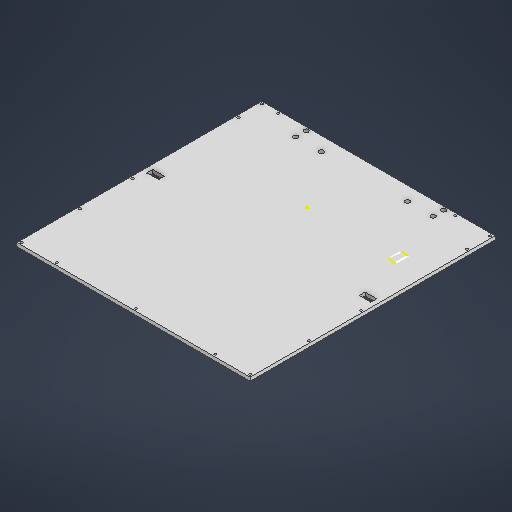
# Autodesk Inventor part: DesignBawahRobot
Saved by Autodesk Inventor 2026.1 (Build 301233020, 233B)
## iProperties
Created: 2025-10-17
Part Number: DesignBawahRobot
Material: Generic
Document SubType Name: Modeling
Designer: FrianVex
Density: 1 g/cm^3
Appearance: Default
Author: FrianVex
Autodesk Inventor part; units mm, degrees
ref_plane "YZ Plane" through (0, 0, 0) normal (1, 0, 0) x (0, 1, 0)
ref_plane "XZ Plane" through (0, 0, 0) normal (0, 1, 0) x (-1, 0, 0)
ref_plane "XY Plane" through (0, 0, 0) normal (0, 0, 1) x (1, 0, 0)
sketch "Sketch1" plane through (0, 0, 0) normal (0, 1, 0) x (-1, 0, 0)
  line L0 (-101.0152, -60.2536) -> (98.9848, -60.2536)
  line L1 (98.9848, -60.2536) -> (98.9848, 149.7464)
  line L2 (98.9848, 149.7464) -> (-101.0152, 149.7464)
  line L3 (-101.0152, 149.7464) -> (-101.0152, -60.2536)
  line L4 (-101.0152, -60.2536) -> (98.9848, 149.7464) construction
  line L5 (98.9848, -60.2536) -> (-101.0152, 149.7464) construction
  line L6 (-65.0152, -60.2536) -> (62.9848, -60.2536)
  line L7 (62.9848, -60.2536) -> (62.9848, -45.2536)
  line L8 (62.9848, -45.2536) -> (-65.0152, -45.2536)
  line L9 (-65.0152, -45.2536) -> (-65.0152, -60.2536)
  line L10 (98.9848, -35.2536) -> (76.9848, -35.2536)
  line L11 (76.9848, -35.2536) -> (76.9848, 34.7464)
  line L12 (76.9848, 34.7464) -> (98.9848, 34.7464)
  line L13 (98.9848, 34.7464) -> (98.9848, -35.2536)
  line L14 (-101.0152, -35.2536) -> (-79.0152, -35.2536)
  line L15 (-79.0152, -35.2536) -> (-79.0152, 34.7464)
  line L16 (-79.0152, 34.7464) -> (-101.0152, 34.7464)
  line L17 (-101.0152, 34.7464) -> (-101.0152, -35.2536)
  line L18 (84.9848, 37.2464) -> (94.9848, 37.2464)
  line L19 (94.9848, 37.2464) -> (94.9848, 42.2464)
  line L20 (94.9848, 42.2464) -> (84.9848, 42.2464)
  line L21 (84.9848, 42.2464) -> (84.9848, 37.2464)
  line L22 (84.9848, 37.2464) -> (94.9848, 42.2464) construction
  line L23 (94.9848, 37.2464) -> (84.9848, 42.2464) construction
  line L24 (-97.0152, 37.2464) -> (-87.0152, 37.2464)
  line L25 (-87.0152, 37.2464) -> (-87.0152, 42.2464)
  line L26 (-87.0152, 42.2464) -> (-97.0152, 42.2464)
  line L27 (-97.0152, 42.2464) -> (-97.0152, 37.2464)
  line L28 (-97.0152, 37.2464) -> (-87.0152, 42.2464) construction
  line L29 (-87.0152, 37.2464) -> (-97.0152, 42.2464) construction
  line L30 (-78.5152, 2.7464) -> (-72.5152, 2.7464)
  line L31 (-72.5152, 2.7464) -> (-72.5152, -8.2536)
  line L32 (-72.5152, -8.2536) -> (-78.5152, -8.2536)
  line L33 (-78.5152, -8.2536) -> (-78.5152, 2.7464)
  line L34 (70.4848, 2.7464) -> (76.4848, 2.7464)
  line L35 (76.4848, 2.7464) -> (76.4848, -8.2536)
  line L36 (76.4848, -8.2536) -> (70.4848, -8.2536)
  line L37 (70.4848, -8.2536) -> (70.4848, 2.7464)
  line L38 (-101.0152, 149.7464) -> (-97.0152, 149.7464)
  circle A0 centre (-99.0152, 147.6464) radius 1
  line L39 (-101.0152, -60.2536) -> (-97.0152, -60.2536)
  line L40 (-101.0152, -36.2536) -> (-101.0152, -60.2536)
  circle A1 centre (-99.0152, -58.1536) radius 1
  circle A2 centre (-99.0152, -38.2536) radius 1
  circle A3 centre (-99.0152, 97.6464) radius 1
  circle A4 centre (-99.0152, 52.6464) radius 1
  circle A5 centre (-69.0152, -58.1536) radius 1
  circle A6 centre (96.9848, -58.1536) radius 1
  circle A7 centre (82.9848, -58.1536) radius 1
  circle A8 centre (96.9848, -38.2536) radius 1
  circle A9 centre (96.9848, 52.6464) radius 1
  circle A10 centre (96.9848, 97.6464) radius 1
  circle A11 centre (96.9848, 147.6464) radius 1
  circle A12 centre (66.9848, 147.6464) radius 1
  circle A13 centre (-69.0152, 147.6464) radius 1.0002
  circle A14 centre (-1.0152, 147.6464) radius 1
  point P0 (-1.0152, 44.7464)
  point P1 (89.9848, 39.7464)
  point P2 (-92.0152, 39.7464)
  point P3 (-101.0152, 34.7464)
  point P4 (98.9848, 34.7464)
  point P5 (62.9848, -60.2536)
  point P6 (-90.0152, -35.2536)
  point P7 (87.9848, 34.7464)
  point P8 (-90.0152, 34.7464)
  point P9 (-99.0152, -60.2536)
  point P10 (-99.0152, 149.7464)
  dimension "d22" = 200
  dimension "d23" = 210
  dimension "d24" = 15
  dimension "d25" = 128
  dimension "d26" = 36
  dimension "d27" = 22
  dimension "d28" = 70
  dimension "d29" = 10
  dimension "d30" = 22
  dimension "d31" = 70
  dimension "d32" = 10
  dimension "d33" = 5
  dimension "d34" = 10
  dimension "d35" = 5
  dimension "d58" = 10
  dimension "d70" = 5
  dimension "d71" = 11
  dimension "d72" = 6
  dimension "d73" = 52
  dimension "d74" = 22.5
  dimension "d75" = 6
  dimension "d76" = 11
  dimension "d77" = 52
  dimension "d78" = 22.5
  dimension "d83" = 4
  dimension "d84" = 4
  dimension "d85" = 5
  dimension "d88" = 2
  dimension "d91" = 2
  dimension "d92" = 2
  dimension "d93" = 22
  dimension "d94" = 2.1
  dimension "d95" = 2
  dimension "d96" = 2
  dimension "d97" = 2.1
  dimension "d98" = 2
  dimension "d99" = 50
  dimension "d100" = 2
  dimension "d101" = 95
  dimension "d102" = 2
  dimension "d104" = 2
  dimension "d105" = 2
  dimension "d106" = 2.1
  dimension "d107" = 2.1
  dimension "d108" = 2
  dimension "d109" = 22
  dimension "d112" = 2.1
  dimension "d113" = 16
  dimension "d114" = 2.1
  dimension "d115" = 32
  dimension "d116" = 32
  dimension "d117" = 2.1
  dimension "d118" = 2
  dimension "d119" = 2.1
  dimension "d120" = 100
  dimension "d122" = 2
  dimension "d123" = 2
  dimension "d124" = 2
  dimension "d125" = 2
  dimension "d126" = 2
  dimension "d178" = 32
  dimension "d179" = 50
  dimension "d180" = 95
  constraints: 82 end point, 16 parallel, 15 centre point, 11 midpoint, 10 horizontal, 8 perpendicular, 7 point on line
  measures "d22" distance of L2.end L1.end
  measures "d23" distance of L0.end L1.end
  measures "d24" distance of L7.end L6.end
  measures "d25" distance of L7.end L8.end
  measures "d26" distance of L0.end L6.end
  measures "d27" distance of L11.end L12.end
  measures "d28" distance of L10.end L11.end
  measures "d29" distance from line of L10 L7.end
  measures "d30" distance of L16.end L15.end
  measures "d31" distance of L14.end L15.end
  measures "d32" distance of L20.end L19.end
  measures "d33" distance of L20.end L18.start
  measures "d34" distance of L26.end L25.end
  measures "d35" distance of L24.end L25.end
  measures "d58" vertical distance of L8.end point (-90.015, -35.254)
  measures "d70" vertical distance of point (87.985, 34.746) point (89.985, 39.746)
  measures "d71" distance of L30.end L31.end
  measures "d72" distance of L30.start L30.end
  measures "d73" distance from line of L6 L31.end
  measures "d74" distance from line of L3 L30.start
  measures "d75" distance of L35.end L36.end
  measures "d76" distance of L36.end L34.start
  measures "d77" distance from line of L0 L35.end
  measures "d78" distance from line of L1 L34.end
  measures "d83" distance from line of L1 L19.end
  measures "d84" distance from line of L3 L24.start
  measures "d85" distance from line of L16 point (-92.015, 39.746)
  measures "d88" diameter of A0
  measures "d91" diameter of A1
  measures "d92" diameter of A2
  measures "d93" distance of point (-99.015, -60.254) A2.centre
  measures "d94" distance of point (-99.015, -60.254) A1.centre
  measures "d95" distance from line of L3 A1.centre
  measures "d96" distance from line of L3 A2.centre
  measures "d97" distance of point (-99.015, 149.746) A0.centre
  measures "d98" diameter of A3
  measures "d99" distance of A3.centre A0.centre
  measures "d100" diameter of A4
  measures "d101" distance of A4.centre A0.centre
  measures "d102" diameter of A5
  measures "d104" diameter of A6
  measures "d105" diameter of A7
  measures "d106" distance from line of L0 A6.centre
  measures "d107" distance from line of L0 A7.centre
  measures "d108" diameter of A8
  measures "d109" distance from line of L0 A8.centre
  measures "d112" distance from line of L2 A11.centre
  measures "d113" distance from line of L1 A7.centre
  measures "d114" distance from line of L2 A12.centre
  measures "d115" distance from line of L1 A12.centre
  measures "d116" distance from line of L3 A13.centre
  measures "d117" distance from line of L2 A13.centre
  measures "d118" diameter of A14
  measures "d119" distance from line of L2 A14.centre
  measures "d120" distance from line of L1 A14.centre
  measures "d122" distance from line of L3 A4.centre
  measures "d123" distance from line of L3 A3.centre
  measures "d124" distance from line of L1 A8.centre
  measures "d125" distance from line of L1 A9.centre
  measures "d126" distance from line of L1 A10.centre
  measures "d178" distance from line of L3 A5.centre
  measures "d179" distance of A11.centre A10.centre
  measures "d180" distance of A11.centre A9.centre
extrude "Body" add sketch "Sketch1" along normal blind 3 contours L3 L14 L15 L16 L2 L1 L12 L11 L10 L0 L7 L8 L9
sketch "Sketch3" plane through (0, 3, 0) normal (0, 1, 0) x (1, 0, 0)
  line L0 (65.0152, 60.2536) -> (65.0152, 45.2536) projected
  line L1 (-62.9848, 60.2536) -> (-98.9848, 60.2536) projected
  line L2 (65.0152, 45.2536) -> (-62.9848, 45.2536)
  line L3 (-62.9848, 45.2536) -> (-62.9848, 60.2536)
  line L4 (-62.9848, 60.2536) -> (65.0152, 60.2536)
  line L5 (65.0152, 60.2536) -> (65.0152, 45.2536)
  circle A0 centre (60.0152, 48.2536) radius 2
  circle A1 centre (60.0152, 57.2536) radius 2
  circle A2 centre (38.0152, 48.2536) radius 2
  circle A3 centre (-57.9848, 57.2536) radius 2
  circle A4 centre (-57.9848, 48.2536) radius 2
  circle A5 centre (-35.9848, 48.2536) radius 2
  point P0 (0, 0)
  point P1 (65.0152, 60.2536)
  dimension "d38" = 4
  dimension "d39" = 5
  dimension "d40" = 3
  dimension "d41" = 4
  dimension "d42" = 3
  dimension "d43" = 5
  dimension "d44" = 4
  dimension "d45" = 27
  dimension "d46" = 3
  dimension "d47" = 4
  dimension "d48" = 3
  dimension "d49" = 5
  dimension "d50" = 4
  dimension "d51" = 5
  dimension "d52" = 3
  dimension "d53" = 4
  dimension "d54" = 3
  dimension "d55" = 27
  constraints: 8 end point, 6 centre point, 2 parallel, 1 horizontal, 1 perpendicular
  measures "d38" diameter of A0
  measures "d39" distance from line of L0 A0.centre
  measures "d40" distance from line of L2 A0.centre
  measures "d41" diameter of A1
  measures "d42" distance from line of L4 A1.centre
  measures "d43" distance from line of L0 A1.centre
  measures "d44" diameter of A2
  measures "d45" distance from line of L0 A2.centre
  measures "d46" distance from line of L2 A2.centre
  measures "d47" diameter of A3
  measures "d48" distance from line of L4 A3.centre
  measures "d49" distance from line of L3 A3.centre
  measures "d50" diameter of A4
  measures "d51" distance from line of L3 A4.centre
  measures "d52" distance from line of L2 A4.centre
  measures "d53" diameter of A5
  measures "d54" distance from line of L2 A5.centre
  measures "d55" distance from line of L3 A5.centre
extrude "IRSensor" add sketch "Sketch3" against normal blind 3
sketch "Sketch4" plane through (0, 3, 0) normal (0, 1, 0) x (1, 0, 0)
  line L0 (101.0152, -34.7464) -> (79.0152, -34.7464)
  line L1 (79.0152, -34.7464) -> (79.0152, 35.2536)
  line L2 (79.0152, 35.2536) -> (101.0152, 35.2536)
  line L3 (101.0152, 35.2536) -> (101.0152, -34.7464)
  point P0 (0, 0)
  constraints: 8 end point, 2 parallel, 1 horizontal, 1 perpendicular
extrude "RodaKrMark" add sketch "Sketch4" against normal blind 3
sketch "Sketch5" plane through (0, 3, 0) normal (0, 1, 0) x (1, 0, 0)
  line L0 (-76.9848, 35.2536) -> (-76.9848, -34.7464) projected
  line L1 (-98.9848, 35.2536) -> (-76.9848, 35.2536) projected
  line L2 (-76.9848, -34.7464) -> (-98.9848, -34.7464)
  line L3 (-98.9848, -34.7464) -> (-98.9848, 35.2536)
  line L4 (-98.9848, 35.2536) -> (-76.9848, 35.2536)
  line L5 (-76.9848, 35.2536) -> (-76.9848, -34.7464)
  point P0 (0, 0)
  constraints: 8 end point, 2 parallel, 1 horizontal, 1 perpendicular
extrude "RodaKaMark" add sketch "Sketch5" against normal blind 3
sketch "Sketch6" plane through (0, 3, 0) normal (0, 1, 0) x (1, 0, 0)
  line L0 (78.5152, -2.7464) -> (72.5152, -2.7464) projected
  line L1 (72.5152, 8.2536) -> (78.5152, 8.2536) projected
  line L2 (78.5152, -2.7464) -> (72.5152, -2.7464)
  line L3 (72.5152, -2.7464) -> (72.5152, 8.2536)
  line L4 (72.5152, 8.2536) -> (78.5152, 8.2536)
  line L5 (78.5152, 8.2536) -> (78.5152, -2.7464)
  point P0 (0, 0)
  constraints: 8 end point, 2 parallel, 1 horizontal, 1 perpendicular
extrude "Extrusion5" add sketch "Sketch6" against normal blind 25
sketch "Sketch8" plane through (0, 3, 0) normal (0, 1, 0) x (1, 0, 0)
  line L0 (-76.4848, -2.7464) -> (-76.4848, 8.2536) projected
  line L1 (-76.4848, 8.2536) -> (-70.4848, 8.2536)
  line L2 (-70.4848, 8.2536) -> (-70.4848, -2.7464)
  line L3 (-70.4848, -2.7464) -> (-76.4848, -2.7464)
  line L4 (-76.4848, -2.7464) -> (-76.4848, 8.2536)
  point P0 (0, 0)
  constraints: 8 end point, 2 parallel, 1 horizontal, 1 perpendicular
extrude "Extrusion6" add sketch "Sketch8" against normal blind 25
sketch "Sketch9" plane through (78.5152, 0, 2.7464) normal (1, 0, 0) x (0, 0, -1)
  line L0 (11, 0) -> (11, -22) projected
  line L1 (63, 0) -> (-147, 0) projected
  line L2 (11, -22) -> (0, -22)
  line L3 (0, -22) -> (0, 0)
  line L4 (0, 0) -> (11, 0)
  line L5 (11, 0) -> (11, -22)
  circle A0 centre (5.5, -4.887) radius 1.5
  circle A1 centre (5.5, -15.887) radius 1.5
  point P0 (2.7464, 0)
  dimension "d146" = 11
  dimension "d147" = 3
  dimension "d148" = 3
  dimension "d149" = 11
  constraints: 8 end point, 2 centre point, 2 parallel, 1 coincident, 1 horizontal, 1 perpendicular, 1 point on line
  measures "d146" distance of L3.end L4.end
  measures "d147" diameter of A0
  measures "d148" diameter of A1
  measures "d149" distance of A0.centre A1.centre
hole "BautBawah" at (78.5152, -15.887, -2.7536) direction (-1, 0, 0) diameter 3 end through all
sketch "Sketch10" plane through (78.5152, 0, 2.7464) normal (1, 0, 0) x (0, 0, -1)
  point P0 (2.7464, 0)
  point P1 (5.5237, -4.8856)
hole "Hole2" at (78.5152, -4.8856, -2.7773) direction (-1, 0, 0) diameter 3 end through all
sketch "Sketch11" plane through (78.5152, 0, 2.7464) normal (1, 0, 0) x (0, 0, -1)
  point P0 (2.7464, 0)
  point P1 (5.5357, -4.6342)
hole "Hole3" at (78.5152, -4.6342, -2.7892) direction (-1, 0, 0) diameter 3 end through all
sketch "Sketch12" plane through (78.5152, 0, 2.7464) normal (1, 0, 0) x (0, 0, -1)
  point P0 (2.7464, 0)
  point P1 (5.5238, -4.1202)
hole "Hole4" at (78.5152, -4.1202, -2.7774) direction (-1, 0, 0) diameter 3 end through all
sketch "Sketch13" plane through (78.5152, 0, 2.7464) normal (1, 0, 0) x (0, 0, -1)
  point P0 (2.7464, 0)
  point P1 (5.5033, -3.3695)
hole "Hole5" at (78.5152, -3.3695, -2.7569) direction (-1, 0, 0) diameter 3 end through all
sketch "Sketch14" plane through (78.5152, 0, 2.7464) normal (1, 0, 0) x (0, 0, -1)
  point P0 (2.7464, 0)
  point P1 (5.5284, -2.8201)
hole "Hole6" at (78.5152, -2.8201, -2.782) direction (-1, 0, 0) diameter 3 end through all
body "Solid1"
